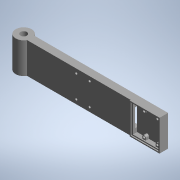
# Autodesk Inventor part: P001-Bras
Saved by Autodesk Inventor 2020 (Build 240168000, 168)
## iProperties
Created: 2021-07-23
Part Number: P001-Bras
Material: Générique
Document SubType Name: Modeling
Designer: gregory.trottet
Density: 1 g/cm^3
Appearance: Par défaut
Author: gregory.trottet
Autodesk Inventor part; units mm, degrees
ref_plane "YZ Plane" through (0, 0, 0) normal (1, 0, 0) x (0, 1, 0)
ref_plane "XZ Plane" through (0, 0, 0) normal (0, 1, 0) x (-1, 0, 0)
ref_plane "XY Plane" through (0, 0, 0) normal (0, 0, 1) x (1, 0, 0)
sketch "Sketch1" plane through (0, 0, 0) normal (0, 0, 1) x (1, 0, 0)
  circle A0 centre (0, 0) radius 3
  arc A1 (6.6332, 3.5) -> (6.6332, -3.5) centre (0, 0) ccw
  line L0 (6.6332, 3.5) -> (131.7417, 3.5)
  line L1 (131.7417, 3.5) -> (131.7417, -4.5)
  line L2 (131.7417, -4.5) -> (103.7417, -4.5)
  line L3 (103.7417, -4.5) -> (103.7417, -3.5)
  line L4 (103.7417, -3.5) -> (6.6332, -3.5)
  line L5 (0, 0) -> (82.0214, 0) construction
  line L6 (3.7417, 6.5) -> (3.7417, -6.5) construction
  line L7 (116.7417, 3.5) -> (116.7417, 8.4968) construction
  line L8 (6.6332, 3.5) -> (6.6332, -3.5) construction
  dimension "d1" = 13
  dimension "d2" = 6
  dimension "d3" = 15
  dimension "d5" = 7
  dimension "d6" = 28
  dimension "d7" = 100
  dimension "d8" = 8
  dimension "d10" = 7.5
  constraints: 18 end point, 4 perpendicular, 4 point on circle, 3 vertical, 2 centre point, 2 coincident, 1 horizontal, 1 parallel, 1 point on line
  measures "d1" distance of L6.start L6.end
  measures "d2" diameter of A0
  measures "d3" distance between parallel lines of L1 L7
  measures "d5" distance between parallel lines of L4 L0
  measures "d6" distance of L1.end L2.end
  measures "d7" distance from line of L6 L2.end
  measures "d8" distance of L0.end L1.end
  measures "d10" radius of A1
extrude "Extrusion1" add sketch "Sketch1" along normal blind 29
sketch "Sketch2" plane through (103.7417, -4.5, 0) normal (0, -1, 0) x (1, 0, 0)
  line L0 (2, 27) -> (26, 27)
  line L1 (26, 27) -> (26, 2)
  line L2 (26, 2) -> (2, 2)
  line L3 (2, 2) -> (2, 27)
  line L4 (0, 29) -> (28, 29) construction
  line L5 (28, 0) -> (28, 29) construction
  line L6 (28, 14.5) -> (26, 14.5) construction
  line L7 (14, 29) -> (14, 27) construction
  circle A0 centre (11.5, 25) radius 1
  circle A1 centre (24, 25) radius 1
  circle A2 centre (24, 4) radius 1
  circle A3 centre (11.5, 4) radius 1
  line L8 (11.5, 25) -> (11.5, 4) construction
  line L9 (11.5, 4) -> (24, 4) construction
  line L10 (24, 4) -> (24, 25) construction
  line L11 (24, 25) -> (11.5, 25) construction
  line L12 (24, 14.5) -> (26, 14.5) construction
  arc A4 (24, 5.6) -> (22.4, 4) centre (24, 4) ccw
  arc A5 (22.4, 25) -> (24, 23.4) centre (24, 25) ccw
  arc A6 (9.9, 25) -> (13.1, 25) centre (11.5, 25) ccw
  arc A7 (13.1, 4) -> (9.9, 4) centre (11.5, 4) ccw
  line L13 (9.9, 4) -> (9.9, 2)
  line L14 (13.1, 4) -> (13.1, 2)
  line L15 (9.9, 25) -> (9.9, 27)
  line L16 (13.1, 25) -> (13.1, 27)
  line L17 (22.4, 25) -> (22.4, 27)
  line L18 (24, 23.4) -> (26, 23.4)
  line L19 (22.4, 4) -> (22.4, 2)
  line L20 (24, 5.6) -> (26, 5.6)
  point P0 (-103.7417, 0)
  dimension "d13" = 25
  dimension "d14" = 24
  dimension "d15" = 21
  dimension "d16" = 12.5
  dimension "d17" = 2
  dimension "d18" = 4
  dimension "d19" = 1.6
  dimension "d20" = 1.6
  constraints: 38 end point, 18 point on line, 11 perpendicular, 8 centre point, 8 point on circle, 5 midpoint, 4 coincident, 3 equal radius, 2 horizontal, 2 parallel, 2 vertical, 1 collinear, 1 vertical alignment
  measures "d13" distance of L0.end L1.end
  measures "d14" distance of L0.start L0.end
  measures "d15" distance of L8.start L8.end
  measures "d16" distance of L10.end L8.start
  measures "d17" diameter of A1
  measures "d18" distance between parallel lines of L5 L10
  measures "d19" radius of A6
  measures "d20" radius of A5
extrude "Extrusion2" cut sketch "Sketch2" against normal blind 5 contours L0 L15 A6 L16 L17 A5 L18 L1 L20 A4 L19 L2 L14 A7 L13 L3
sketch "Sketch3" plane through (103.7417, -4.5, 0) normal (0, -1, 0) x (1, 0, 0)
  line L0 (13.1, 2) -> (13.1, 4) construction
  arc A0 (13.1, 4) -> (9.9, 4) centre (11.5, 4) ccw construction
  line L1 (9.9, 4) -> (9.9, 2) construction
  line L2 (9.9, 2) -> (2, 2) construction
  line L3 (2, 2) -> (2, 27) construction
  line L4 (2, 27) -> (9.9, 27) construction
  line L5 (9.9, 27) -> (9.9, 25) construction
  arc A1 (9.9, 25) -> (13.1, 25) centre (11.5, 25) ccw construction
  line L6 (13.1, 25) -> (13.1, 27) construction
  line L7 (13.1, 27) -> (22.4, 27) construction
  line L8 (22.4, 27) -> (22.4, 25) construction
  arc A2 (22.4, 25) -> (24, 23.4) centre (24, 25) ccw construction
  line L9 (24, 23.4) -> (26, 23.4) construction
  line L10 (26, 23.4) -> (26, 5.6) construction
  line L11 (26, 5.6) -> (24, 5.6) construction
  arc A3 (24, 5.6) -> (22.4, 4) centre (24, 4) ccw construction
  line L12 (22.4, 4) -> (22.4, 2) construction
  line L13 (22.4, 2) -> (13.1, 2) construction
  line L14 (0, 0) -> (28, 0) construction
  line L15 (28, 0) -> (28, 29) construction
  line L16 (0, 29) -> (28, 29) construction
  line L17 (0, 0) -> (0, 29) construction
  line L18 (1, 28) -> (27, 28)
  line L19 (27, 28) -> (27, 1)
  line L20 (27, 1) -> (1, 1)
  line L21 (1, 1) -> (1, 28)
  line L22 (28, 14.5) -> (27, 14.5) construction
  line L23 (14, 1) -> (14, 0) construction
  point P0 (-103.7417, 0)
  dimension "d23" = 26
  dimension "d24" = 27
  constraints: 12 end point, 4 midpoint, 2 horizontal, 2 parallel, 1 perpendicular, 1 vertical
  measures "d23" distance between parallel lines of L21 L19
  measures "d24" distance of L18.end L19.end
extrude "Extrusion3" cut sketch "Sketch3" against normal blind 1
sketch "Sketch4" plane through (103.7417, -3.5, 0) normal (0, -1, 0) x (1, 0, 0)
  line L0 (13.1, 4) -> (13.1, 2) construction
  arc A0 (13.1, 4) -> (9.9, 4) centre (11.5, 4) ccw construction
  line L1 (9.9, 2) -> (9.9, 4) construction
  line L2 (2, 2) -> (9.9, 2) construction
  line L3 (2, 27) -> (2, 2) construction
  line L4 (9.9, 27) -> (2, 27) construction
  line L5 (9.9, 25) -> (9.9, 27) construction
  arc A1 (9.9, 25) -> (13.1, 25) centre (11.5, 25) ccw construction
  line L6 (13.1, 27) -> (13.1, 25) construction
  line L7 (22.4, 27) -> (13.1, 27) construction
  line L8 (22.4, 25) -> (22.4, 27) construction
  arc A2 (22.4, 25) -> (24, 23.4) centre (24, 25) ccw construction
  line L9 (26, 23.4) -> (24, 23.4) construction
  line L10 (26, 5.6) -> (26, 23.4) construction
  line L11 (24, 5.6) -> (26, 5.6) construction
  arc A3 (24, 5.6) -> (22.4, 4) centre (24, 4) ccw construction
  line L12 (22.4, 2) -> (22.4, 4) construction
  line L13 (13.1, 2) -> (22.4, 2) construction
  line L14 (1, 28) -> (27, 28) construction
  line L15 (1, 1) -> (1, 28) construction
  line L16 (27, 1) -> (1, 1) construction
  line L17 (27, 28) -> (27, 1) construction
  circle A4 centre (11.5, 25) radius 1
  circle A5 centre (24, 25) radius 1
  circle A6 centre (24, 4) radius 1
  circle A7 centre (11.5, 4) radius 1
  point P0 (-103.7417, 0)
  dimension "d27" = 2
  constraints: 4 centre point, 4 coincident, 3 equal radius
  measures "d27" diameter of A4
extrude "Extrusion4" cut sketch "Sketch4" against normal through all
sketch "Sketch5" plane through (6.6332, 3.5, 0) normal (0, 1, 0) x (1, 0, 0)
  line L0 (0.2, -6) -> (99.1084, -6)
  line L1 (99.1084, -6) -> (99.1084, -23)
  line L2 (99.1084, -23) -> (0.2, -23)
  line L3 (0.2, -23) -> (0.2, -6)
  line L4 (0, 0) -> (0, 0) construction
  line L5 (0, 0) -> (0, -29) construction
  line L6 (0, -29) -> (0, -29) construction
  line L7 (0, 0) -> (0, -29) construction
  line L8 (0, -14.5) -> (0.2, -14.5) construction
  line L9 (125.1084, 0) -> (125.1084, -29) construction
  point P0 (-6.6332, 0)
  dimension "d30" = 17
  dimension "d31" = 26
  dimension "d32" = 0.2
  constraints: 10 end point, 2 horizontal, 2 midpoint, 2 parallel, 1 perpendicular
  measures "d30" distance of L0.end L1.end
  measures "d31" distance between parallel lines of L9 L1
  measures "d32" distance of L8.start L8.end
extrude "Extrusion5" cut sketch "Sketch5" against normal blind 2.5
sketch "Sketch6" plane through (6.6332, 3.5, 0) normal (0, 1, 0) x (1, 0, 0)
  line L0 (8.1084, -4.75) -> (100.1084, -4.75)
  line L1 (100.1084, -4.75) -> (100.1084, -24.25)
  line L2 (100.1084, -24.25) -> (8.1084, -24.25)
  line L3 (8.1084, -24.25) -> (8.1084, -4.75)
  line L4 (97.1084, 0) -> (97.1084, -29) construction
  line L5 (97.1084, -14.5) -> (100.1084, -14.5) construction
  line L6 (125.1084, 0) -> (125.1084, -29) construction
  point P0 (-6.6332, 0)
  dimension "d36" = 92
  dimension "d37" = 19.5
  dimension "d52" = 25
  constraints: 10 end point, 2 horizontal, 2 midpoint, 2 parallel, 1 perpendicular
  measures "d36" distance of L0.start L0.end
  measures "d37" distance of L0.end L1.end
  measures "d52" distance between parallel lines of L6 L1
extrude "Extrusion6" cut sketch "Sketch6" against normal blind 0.5
fillet "Fillet3" radius 5 1 edges at (6.8332, 3.5, 14.5)
fillet "Fillet4" radius 5 1 edges at (6.8332, 1, 14.5)
sketch "Sketch10" plane through (6.6332, 1, 0) normal (0, 1, 0) x (1, 0, 0)
  line L0 (4.3301, -23) -> (4.3301, -6) construction
  line L1 (99.1084, -23) -> (4.3301, -23) construction
  line L2 (99.1084, -6) -> (99.1084, -23) construction
  line L3 (4.3301, -6) -> (99.1084, -6) construction
  line L4 (99.1084, -6) -> (91.1084, -6)
  line L5 (91.1084, -6) -> (91.1084, -23)
  line L6 (91.1084, -23) -> (99.1084, -23)
  line L7 (99.1084, -23) -> (99.1084, -6)
  point P0 (-6.6332, 0)
  dimension "d55" = 8
  constraints: 8 end point, 2 parallel, 1 horizontal, 1 perpendicular, 1 point on line
  measures "d55" distance between parallel lines of L2 L5
extrude "Extrusion10" cut sketch "Sketch10" against normal blind 2.5
chamfer "Chamfer1" distance 10 distance2 2.5 1 edges at (97.7417, 1, 14.5) measured on face at (39.8895, 1, 11.6667)
sketch "Sketch11" plane through (6.6332, 3.5, 0) normal (0, 1, 0) x (1, 0, 0)
  line L0 (58.6084, -25) -> (46.1084, -25)
  line L1 (46.1084, -25) -> (46.1084, -4)
  line L2 (46.1084, -4) -> (58.6084, -4)
  line L3 (58.6084, -4) -> (58.6084, -25)
  line L4 (125.1084, -29) -> (0, -29) construction
  circle A0 centre (108.6084, -4) radius 1 construction
  circle A1 centre (108.6084, -25) radius 1 construction
  circle A2 centre (121.1084, -4) radius 1 construction
  circle A3 centre (121.1084, -25) radius 1 construction
  line L5 (0, -23) -> (8.1084, -23) construction
  line L6 (0, -23) -> (0, -29) construction
  line L7 (125.1084, -29) -> (0, -29) construction
  line L8 (125.1084, 0) -> (125.1084, -29) construction
  line L9 (125.1084, 0) -> (0, 0) construction
  line L10 (0, 0) -> (0, -6) construction
  line L11 (8.1084, -6) -> (0, -6) construction
  line L12 (8.1084, -6) -> (8.1084, -4.75) construction
  line L13 (8.1084, -4.75) -> (100.1084, -4.75) construction
  line L14 (100.1084, -4.75) -> (100.1084, -24.25) construction
  line L15 (100.1084, -24.25) -> (8.1084, -24.25) construction
  line L16 (8.1084, -24.25) -> (8.1084, -23) construction
  line L17 (100.1084, -14.5) -> (58.6084, -14.5)
  point P0 (-6.6332, 0)
  dimension "d68" = 21
  dimension "d69" = 12.5
  dimension "d71" = 50
  constraints: 10 end point, 3 horizontal, 2 midpoint, 2 vertical
  measures "d68" distance of L2.end L0.start
  measures "d69" distance of L0.start L0.end
  measures "d71" distance from line of A0.centre L3
hole "Hole1" at (65.2417, 3.5, 25) at (52.7417, 3.5, 25) at (65.2417, 3.5, 4) at (52.7417, 3.5, 4) direction (0, -1, 0) diameter 2 depth 17.1 tip angle 118
sketch "Sketch14" plane through (103.7417, -3.5, 0) normal (0, -1, 0) x (1, 0, 0)
  circle A0 centre (24, 25) radius 1 projected
  circle A1 centre (24, 4) radius 1 construction
  circle A2 centre (11.5, 25) radius 1 projected
  circle A3 centre (11.5, 4) radius 1 projected
  line L0 (13.1, 4) -> (13.1, 2) projected
  arc A4 (13.1, 4) -> (9.9, 4) centre (11.5, 4) ccw projected
  line L1 (9.9, 2) -> (9.9, 4) projected
  line L2 (2, 2) -> (9.9, 2) construction
  line L3 (2, 27) -> (2, 2) construction
  line L4 (9.9, 27) -> (2, 27) construction
  line L5 (9.9, 25) -> (9.9, 27) projected
  arc A5 (9.9, 25) -> (13.1, 25) centre (11.5, 25) ccw projected
  line L6 (13.1, 27) -> (13.1, 25) projected
  line L7 (22.4, 27) -> (13.1, 27) construction
  line L8 (22.4, 25) -> (22.4, 27) projected
  arc A6 (22.4, 25) -> (24, 23.4) centre (24, 25) ccw projected
  line L9 (26, 23.4) -> (24, 23.4) projected
  line L10 (26, 5.6) -> (26, 23.4) construction
  line L11 (24, 5.6) -> (26, 5.6) projected
  arc A7 (24, 5.6) -> (22.4, 4) centre (24, 4) ccw projected
  line L12 (22.4, 2) -> (22.4, 4) projected
  line L13 (13.1, 2) -> (22.4, 2) construction
  line L14 (1, 1) -> (1, 28) construction
  line L15 (27, 1) -> (1, 1) construction
  line L16 (27, 28) -> (27, 1) construction
  line L17 (1, 28) -> (27, 28) construction
  line L18 (9.9, 27) -> (2, 27) construction
  line L19 (9.9, 27) -> (13.1, 27)
  line L20 (28, 29) -> (-97.1084, 29) construction
  line L21 (22.4, 27) -> (13.1, 27) construction
  line L22 (22.4, 27) -> (26, 27)
  line L23 (26, 27) -> (26, 23.4)
  line L24 (26, 5.6) -> (26, 2)
  line L25 (26, 2) -> (22.4, 2)
  line L26 (9.9, 2) -> (2, 2) construction
  line L27 (13.1, 4) -> (13.1, 2) projected
  line L28 (9.9, 2) -> (13.1, 2)
  point P0 (-103.7417, 0)
  constraints: 12 end point, 2 perpendicular, 1 horizontal, 1 parallel, 1 point on line, 1 vertical
extrude "Extrusion11" cut sketch "Sketch14" against normal blind 1
body "Solid1"
